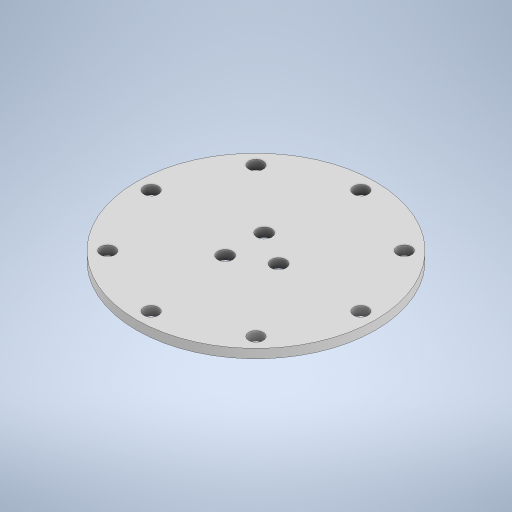
# Autodesk Inventor part: Bell_KoloFormaDol
Saved by Autodesk Inventor 2023 (Build 270158000, 158)
## iProperties
Created: 2023-05-03
Part Number: Bell_KoloFormaDol
Material: Ogólny
Document SubType Name: Modeling
Designer: julia
Density: 1 g/cm^3
Appearance: Domyślna
Author: julia
Autodesk Inventor part; units mm, degrees
ref_plane "YZ Plane" through (0, 0, 0) normal (1, 0, 0) x (0, 1, 0)
ref_plane "XZ Plane" through (0, 0, 0) normal (0, 1, 0) x (-1, 0, 0)
ref_plane "XY Plane" through (0, 0, 0) normal (0, 0, 1) x (1, 0, 0)
sketch "Szkic1" plane through (0, 0, 0) normal (0, 1, 0) x (-1, 0, 0)
  circle A0 centre (0, 0) radius 20
  circle A1 centre (0, 0) radius 26.5
  line L0 (0, 26.5) -> (0, 20)
  circle A2 centre (0, 23.25) radius 1.6
  circle A3 centre (-16.4402, 16.4402) radius 1.6
  circle A4 centre (-23.25, 0) radius 1.6
  circle A5 centre (-16.4402, -16.4402) radius 1.6
  circle A6 centre (0, -23.25) radius 1.6
  circle A7 centre (16.4402, -16.4402) radius 1.6
  circle A8 centre (23.25, 0) radius 1.6
  circle A9 centre (16.4402, 16.4402) radius 1.6
  dimension "d0" = 40
  dimension "d1" = 53
  dimension "d2" = 3.2
  dimension "d5" = 360
  constraints: 10 coincident, 8 centre point, 2 end point, 2 vertical alignment, 1 midpoint, 1 vertical, 29 other
  measures "d2" diameter of A2
extrude "Wyciągnięcie proste1" add sketch "Szkic1" along normal blind 2 contours A0 | A1
sketch "Szkic3" plane through (0, 2, 0) normal (0, 1, 0) x (1, 0, 0)
  circle A0 centre (0, 0) radius 5
  circle A1 centre (5, 0) radius 1.65
  circle A2 centre (-2.5, 4.3301) radius 1.65
  circle A3 centre (-2.5, -4.3301) radius 1.65
  point P0 (1.5451, -4.7553)
  point P1 (1.5451, 4.7553)
  point P2 (-4.0451, 2.9389)
  dimension "d22" = 10
  dimension "d39" = 3.3
  dimension "d42" = 360
  constraints: 4 centre point, 3 coincident, 7 other
  measures "d22" diameter of A0
  measures "d39" diameter of A1
hole "Otwór2" at (5, 2, 0) at (-2.5, 2, -4.3301) at (-2.5, 2, 4.3301) direction (0, -1, 0) diameter 3.3 end through all
